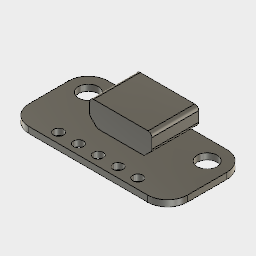
1833 micro USB Breakout (Autodesk Fusion 360 design; units mm, degrees)
Autodesk Fusion 360 part; units mm, degrees
note: some values were not read from the file. Set by a fixed rule: which sketch regions a step uses.
sketch "Sketch1" plane through (0, 0, 0) normal (0, 0, 1) x (1, 0, 0)
  line L0 (6.86, 8.042) -> (6.86, 7.442)
  arc A0 (17.78, 0) -> (20.32, 2.54) centre (17.78, 2.54) ccw
  arc A1 (13.76, 8.292) -> (13.46, 8.042) centre (13.735, 8.017) ccw
  line L1 (13.46, 7.442) -> (13.46, 8.042)
  line L2 (14.06, 8.042) -> (14.06, 7.442)
  arc A2 (14.06, 8.042) -> (13.76, 8.292) centre (13.785, 8.017) ccw
  arc A3 (6.86, 8.042) -> (6.56, 8.292) centre (6.585, 8.017) ccw
  arc A4 (6.56, 7.192) -> (6.86, 7.442) centre (6.585, 7.467) ccw
  line L3 (6.26, 7.442) -> (6.26, 8.042)
  arc A5 (6.26, 7.442) -> (6.56, 7.192) centre (6.535, 7.467) ccw
  line L4 (2.54, 10.16) -> (17.78, 10.16)
  line L5 (17.78, 0) -> (2.54, 0)
  line L6 (0, 2.54) -> (0, 7.62)
  arc A6 (13.76, 7.192) -> (14.06, 7.442) centre (13.785, 7.467) ccw
  arc A7 (2.54, 10.16) -> (0, 7.62) centre (2.54, 7.62) ccw
  arc A8 (0, 2.54) -> (2.54, 0) centre (2.54, 2.54) ccw
  line L7 (20.32, 7.62) -> (20.32, 2.54)
  arc A9 (13.46, 7.442) -> (13.76, 7.192) centre (13.735, 7.467) ccw
  arc A10 (20.32, 7.62) -> (17.78, 10.16) centre (17.78, 7.62) ccw
  arc A11 (6.56, 8.292) -> (6.26, 8.042) centre (6.535, 8.017) ccw
  line L8 (4.191, 2.159) -> (4.191, 0.381)
  arc A12 (17.78, 6.741) -> (17.78, 8.499) centre (17.78, 7.62) ccw
  line L9 (7.81, 8.992) -> (5.31, 8.992)
  line L10 (12.51, 8.992) -> (12.51, 6.492)
  arc A13 (17.78, 8.499) -> (17.78, 6.741) centre (17.78, 7.62) ccw
  line L11 (15.01, 6.492) -> (15.01, 8.992)
  arc A14 (17.78, 6.741) -> (17.78, 8.499) centre (17.78, 7.62) ccw
  arc A15 (17.78, 8.499) -> (17.78, 6.741) centre (17.78, 7.62) ccw
  line L12 (7.81, 8.992) -> (5.31, 8.992)
  line L13 (5.969, 2.159) -> (4.191, 2.159)
  arc A16 (2.54, 6.741) -> (2.54, 8.499) centre (2.54, 7.62) ccw
  line L14 (4.191, 0.381) -> (5.969, 0.381)
  line L15 (5.969, 0.381) -> (5.969, 2.159)
  arc A17 (2.54, 6.741) -> (2.54, 8.499) centre (2.54, 7.62) ccw
  line L16 (4.191, 0.381) -> (5.969, 0.381)
  line L17 (12.51, 8.992) -> (12.51, 6.492)
  line L18 (5.31, 6.492) -> (7.81, 6.492)
  line L19 (5.31, 8.992) -> (5.31, 6.492)
  line L20 (4.191, 2.159) -> (4.191, 0.381)
  line L21 (7.81, 6.492) -> (7.81, 8.992)
  line L22 (12.51, 6.492) -> (15.01, 6.492)
  line L23 (5.31, 8.992) -> (5.31, 6.492)
  line L24 (7.81, 6.492) -> (7.81, 8.992)
  line L25 (15.01, 6.492) -> (15.01, 8.992)
  line L26 (15.01, 8.992) -> (12.51, 8.992)
  line L27 (12.51, 6.492) -> (15.01, 6.492)
  line L28 (15.01, 8.992) -> (12.51, 8.992)
  arc A18 (2.54, 8.499) -> (2.54, 6.741) centre (2.54, 7.62) ccw
  line L29 (5.31, 6.492) -> (7.81, 6.492)
  line L30 (5.969, 0.381) -> (5.969, 2.159)
  arc A19 (2.54, 8.499) -> (2.54, 6.741) centre (2.54, 7.62) ccw
  line L31 (5.969, 2.159) -> (4.191, 2.159)
  circle A20 centre (2.54, 7.62) radius 1.27
  circle A21 centre (17.78, 7.62) radius 1.27
  circle A22 centre (5.08, 1.27) radius 0.635
  circle A23 centre (7.62, 1.27) radius 0.635
  circle A24 centre (10.16, 1.27) radius 0.635
  circle A25 centre (12.7, 1.27) radius 0.635
  circle A26 centre (15.24, 1.27) radius 0.635
  dimension "d5" = 2.54
  dimension "d6" = 2.54
  dimension "d9" = 1.27
  dimension "d12" = 2.54
  dimension "d13" = 0
  measures "d5" diameter of A20
  measures "d6" diameter of A21
  measures "d9" diameter of A22
extrude "Extrude1" add sketch "Sketch1" along normal blind 0.8 contours L0 A3 A4 L3 A5 A11 | A0 L4 L5 L6 A7 A8 L7 A10 | A1 L1 L2 A2 A6 A9 | L8 L13 L14 L15 L16 L20 L30 L31 | L9 L12 L18 L19 L21 L23 L24 L29 | L10 L11 L17 L22 L25 L26 L27 L28 makes body 1
sketch "Sketch2" plane through (0, 0, 0.8) normal (0, 0, 1) x (-1, 0, 0)
  circle A0 centre (-7.62, -1.27) radius 0.635
  circle A1 centre (-15.24, -1.27) radius 0.635
  circle A2 centre (-2.54, -7.62) radius 1.27
  circle A3 centre (-17.78, -7.62) radius 1.27
  circle A4 centre (-5.08, -1.27) radius 0.635
  circle A5 centre (-12.7, -1.27) radius 0.635
  circle A6 centre (-10.16, -1.27) radius 0.635
  arc A7 (-17.78, 0) -> (-20.32, -2.54) centre (-17.78, -2.54) ccw
  line L0 (-20.32, -2.54) -> (-20.32, -7.62)
  arc A8 (-20.32, -7.62) -> (-17.78, -10.16) centre (-17.78, -7.62) ccw
  line L1 (-17.78, -10.16) -> (-2.54, -10.16)
  arc A9 (-2.54, -10.16) -> (0, -7.62) centre (-2.54, -7.62) ccw
  line L2 (0, -7.62) -> (0, -2.54)
  arc A10 (0, -2.54) -> (-2.54, 0) centre (-2.54, -2.54) ccw
  line L3 (-2.54, 0) -> (-17.78, 0)
  line L4 (-6.16, -10.16) -> (-14.16, -10.16)
  line L5 (-14.16, -10.16) -> (-14.16, -4.16)
  line L6 (-14.16, -4.16) -> (-6.16, -4.16)
  line L7 (-6.16, -4.16) -> (-6.16, -10.16)
  line L8 (-6.16, -10.16) -> (-14.16, -4.16) construction
  line L9 (-14.16, -10.16) -> (-6.16, -4.16) construction
  point P0 (-10.16, -7.16)
  dimension "d14" = 6
  dimension "d15" = 8
  measures "d14" distance of L4.end L5.end
  measures "d15" distance of L5.end L6.end
extrude "Extrude2" add sketch "Sketch2" along normal blind 3 separate body contours L1 L4 L5 L6 L7 makes body 2
chamfer "Chamfer1" distance 1 angle 45 2 edges at (14.16, 7.16, 0.8) (6.16, 7.16, 0.8) on bodies 2
fillet "Fillet1" radius 0.5 6 edges at (6.16, 7.16, 3.8) (6.16, 7.16, 1.8) (7.16, 7.16, 0.8) (13.16, 7.16, 0.8) (14.16, 7.16, 1.8) (14.16, 7.16, 3.8) on bodies 2
shell "Shell1" thickness 0.4 removed faces 1 at (11.091, 10.16, 2.8) on bodies 2
